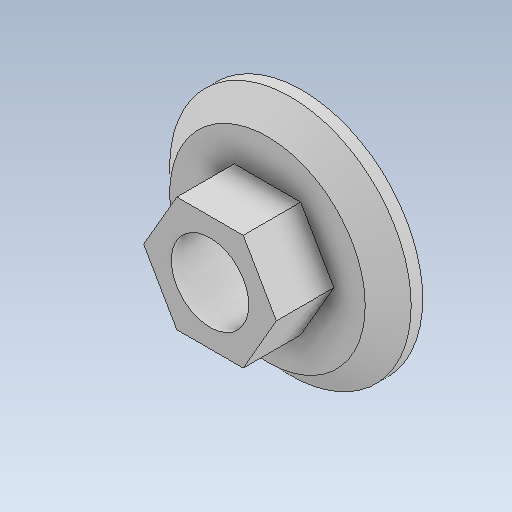
# Autodesk Inventor part: Tuerca para tornillo
Saved by Autodesk Inventor 2021 (Build 250183000, 183)
## iProperties
Created: 2020-11-09
Part Number: Tuerca para tornillo
Material: Genérico
Document SubType Name: Modeling
Designer: juanm
Density: 1 g/cm^3
Appearance: Valor por defecto
Author: juanm
Autodesk Inventor part; units mm, degrees
ref_plane "YZ Plane" through (0, 0, 0) normal (1, 0, 0) x (0, 1, 0)
ref_plane "XZ Plane" through (0, 0, 0) normal (0, 1, 0) x (-1, 0, 0)
ref_plane "XY Plane" through (0, 0, 0) normal (0, 0, 1) x (1, 0, 0)
sketch "Boceto1" plane through (0, 0, 0) normal (0, 0, 1) x (1, 0, 0)
  point P0 (0, 0)
sketch "Boceto2" plane through (0, 0, 0) normal (0, 0, 1) x (1, 0, 0)
  circle A0 centre (0, 0) radius 10.5
  dimension "d0" = 21
  constraints: 1 centre point, 1 coincident
  measures "d0" diameter of A0
extrude "Extrusión1" add sketch "Boceto2" along normal blind 1
sketch "Boceto3" plane through (0, 0, 1) normal (0, 0, 1) x (1, 0, 0)
  circle A0 centre (0, 0) radius 3.375
  circle A1 centre (0, 0) radius 5
  line L0 (0, 5) -> (3, 5)
  line L1 (0, 8.6714) -> (0, 6.7493)
  line L2 (0, 5) -> (-3, 5)
  line L3 (-4.3301, 2.5) -> (-2.8301, 5.0981)
  line L4 (-4.3301, 2.5) -> (-5.8301, -0.0981)
  line L5 (-4.3301, -2.5) -> (-5.8301, 0.0981)
  line L6 (-4.3301, -2.5) -> (-2.8301, -5.0981)
  line L7 (0, -5) -> (-3, -5)
  line L8 (0, -5) -> (3, -5)
  line L9 (4.3301, -2.5) -> (2.8301, -5.0981)
  line L10 (4.3301, -2.5) -> (5.8301, 0.0981)
  line L11 (4.3301, 2.5) -> (5.8301, -0.0981)
  line L12 (4.3301, 2.5) -> (2.8301, 5.0981)
  point P0 (-2.8868, 5)
  point P1 (-5.7735, 0)
  point P2 (-2.8868, -5)
  point P3 (2.8868, -5)
  point P4 (5.7735, 0)
  point P5 (2.8868, 5)
  dimension "d4" = 10
  dimension "d3" = 6.75
  dimension "d5" = 3
  dimension "d8" = 360
  constraints: 26 end point, 2 coincident, 2 horizontal, 1 centre point, 1 symmetric about line, 1 vertical, 1 vertical alignment, 33 other
  measures "d3" diameter of A0
  measures "d5" distance of L0.start L0.end
extrude "Extrusión2" add sketch "Boceto3" along normal blind 7
sketch "Boceto4" plane through (0, 0, 1) normal (0, 0, 1) x (1, 0, 0)
  circle A0 centre (0, 0) radius 10.5
  constraints: 1 centre point, 1 coincident
extrude "Extrusión3" add sketch "Boceto4" along normal blind 2
chamfer "Chaflán1" distance 2 angle 45 1 edges at (-10.5, 0, 3)
sketch "Boceto5" plane through (0, 0, 8) normal (0, 0, 1) x (1, 0, 0)
  circle A0 centre (0, 0) radius 3.375
  constraints: 1 centre point, 1 coincident
extrude "Extrusión4" cut sketch "Boceto5" against normal blind 8
